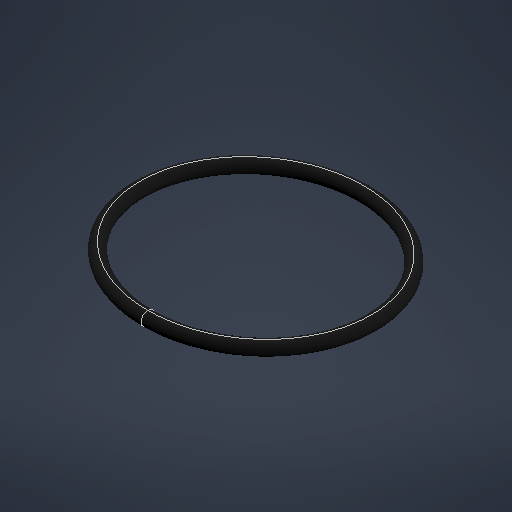
# Autodesk Inventor part: BEARING_SPACERS_CORE,REV-ENG
Saved by Autodesk Inventor 2026.2 (Build 302298010, 298A)
## iProperties
Created: 2026-03-06
Part Number: BEARING_SPACERS_CORE,REV-ENG
Material: Polyethylene, UHMW
Document SubType Name: Modeling
Designer: 4aida
Density: 0.930045 g/cm^3
Appearance: Black
Author: 4aida
Autodesk Inventor part; units mm, degrees
ref_plane "YZ Plane" through (0, 0, 0) normal (1, 0, 0) x (0, 1, 0)
ref_plane "XZ Plane" through (0, 0, 0) normal (0, 1, 0) x (-1, 0, 0)
ref_plane "XY Plane" through (0, 0, 0) normal (0, 0, 1) x (1, 0, 0)
sketch "Sketch1" plane through (0, 0, 0) normal (0, 1, 0) x (-1, 0, 0)
  ellipse E0 centre (0, 0) end of major axis (0, 13.95) minor radius 14.95
  dimension "d0" = 14.95
  dimension "d1" = 13.95
  constraints: 1 coincident, 2 other
sketch "Sketch2" plane through (0, 0, 0) normal (1, 0, 0) x (0, 1, 0)
  circle A0 centre (0, 13.95) radius 0.875
  point P0 (0, 0)
  dimension "d2" = 1.75
  dimension "d3" = 13.95
  constraints: 1 centre point, 1 vertical alignment
  measures "d2" diameter of A0
  measures "d3" distance of point (0, 0) A0.centre
sweep "Sweep1" add profiles "Sketch2" path "Sketch1"
equation "\"d3\" = d1"
body "Solid1"
